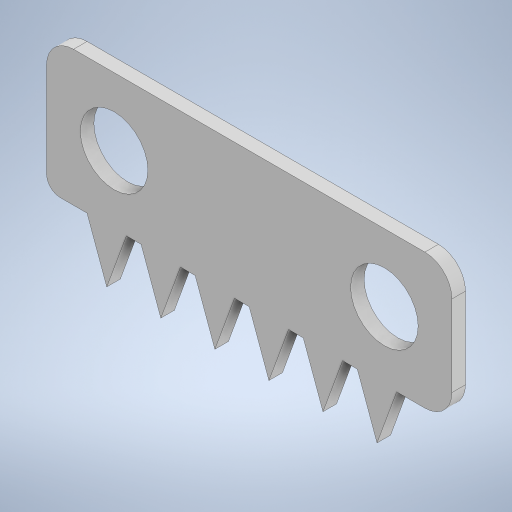
# Autodesk Inventor part: 50_sierra-01
Saved by Autodesk Inventor 2023.2 (Build 272271030, 271C)
## iProperties
Created: 2023-07-12
Part Number: 50_sierra-01
Material: Generic
Document SubType Name: Modeling
Designer: Cris Pat
Density: 1 g/cm^3
Appearance: Default
Author: Cris Pat
Autodesk Inventor part; units mm, degrees
ref_plane "YZ Plane" through (0, 0, 0) normal (1, 0, 0) x (0, 1, 0)
ref_plane "XZ Plane" through (0, 0, 0) normal (0, 1, 0) x (-1, 0, 0)
ref_plane "XY Plane" through (0, 0, 0) normal (0, 0, 1) x (1, 0, 0)
sketch "Sketch2" plane through (0, 0, 0) normal (0, 0, 1) x (1, 0, 0)
  line L0 (15, -5) -> (-15, -5)
  line L1 (-15, -5) -> (-15, 5)
  line L2 (-15, 5) -> (15, 5)
  line L3 (15, 5) -> (15, -5)
  line L4 (15, -5) -> (-15, 5) construction
  line L5 (-15, -5) -> (15, 5) construction
  point P0 (0, 0)
  dimension "d192" = 30
  dimension "d193" = 10
  constraints: 12 end point, 2 midpoint, 2 parallel, 1 horizontal, 1 perpendicular
  measures "d192" distance of L1.end L2.end
  measures "d193" distance of L0.end L1.end
extrude "Extrusion1" add sketch "Sketch2" along normal blind 1
sketch "Sketch3" plane through (0, 0, 1) normal (0, 0, 1) x (1, 0, 0)
  circle A0 centre (-10, 0) radius 2.5
  line L0 (15, 5) -> (-15, 5) construction
  line L1 (-15, 5) -> (-15, -5) construction
  line L2 (-15, -5) -> (15, -5) construction
  line L3 (15, -5) -> (15, 5) construction
  point P0 (0, 0)
  dimension "d196" = 5
  dimension "d197" = 10
  constraints: 1 centre point, 1 horizontal alignment
  measures "d196" diameter of A0
  measures "d197" distance of A0.centre point (0, 0)
extrude "Extrusion2" cut sketch "Sketch3" against normal blind 1
sketch "Sketch4" plane through (0, 0, 1) normal (0, 0, 1) x (1, 0, 0)
  circle A0 centre (10, 0) radius 2.5
  point P0 (0, 0)
  dimension "d200" = 5
  dimension "d201" = 10
  constraints: 1 centre point, 1 horizontal alignment
  measures "d200" diameter of A0
  measures "d201" distance of A0.centre point (0, 0)
extrude "Extrusion3" cut sketch "Sketch4" against normal blind 1
sketch "Sketch5" plane through (0, 0, 1) normal (0, 0, 1) x (1, 0, 0)
  line L0 (-15, -5) -> (15, -5) construction
  line L1 (-15, -5) -> (15, -5) projected
  line L2 (-12, -5) -> (-10.5441, -9)
  line L3 (-10.5441, -9) -> (-9.0882, -5)
  point P0 (0, 0)
  dimension "d204" = 4
  dimension "d205" = 70
  dimension "d206" = 70
  dimension "d207" = 12
  constraints: 4 end point, 2 point on line
  measures "d204" distance from line of L0 L2.end
  measures "d205" angle of L0 L2
  measures "d206" angle of L3 L0
  measures "d207" horizontal distance of point (0, 0) L2.start
extrude "Extrusion4" add sketch "Sketch5" against normal blind 1
pattern_linear "Rectangular Pattern1" count 6 spacing 4 along (1, 0, 0) of "Extrusion4"
fillet "Fillet1" radius 2 1 edges at (-15, 5, 0.5)
fillet "Fillet2" radius 2 1 edges at (15, 5, 0.5)
fillet "Fillet3" radius 2 1 edges at (15, -5, 0.5)
fillet "Fillet4" radius 1 1 edges at (-15, -5, 0.5)
body "Solid1"
